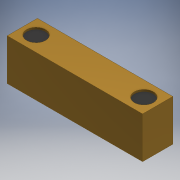
# Autodesk Inventor part: Camera
Saved by Autodesk Inventor 2018 (Build 220112000, 112)
## iProperties
Created: 2018-03-27
Part Number: Camera
Material: Brass, Soft Yellow
Document SubType Name: Modeling
Designer: JARVIS
Mass: 2221.17 g
Surface Area: 296.985 cm^2
Volume: 262.239 cm^3
Density: 8.47 g/cm^3
Appearance: Brass - Satin
Author: JARVIS
Autodesk Inventor part; units mm, degrees
ref_plane "YZ Plane" through (0, 0, 0) normal (1, 0, 0) x (0, 1, 0)
ref_plane "XZ Plane" through (0, 0, 0) normal (0, 1, 0) x (-1, 0, 0)
ref_plane "XY Plane" through (0, 0, 0) normal (0, 0, 1) x (1, 0, 0)
sketch "Sketch1" plane through (0, 0, 0) normal (0, 0, 1) x (1, 0, 0)
  line L0 (-78.5, 17.5) -> (78.5, 17.5)
  line L1 (78.5, 17.5) -> (78.5, -17.5)
  line L2 (78.5, -17.5) -> (-78.5, -17.5)
  line L3 (-78.5, -17.5) -> (-78.5, 17.5)
  point P0 (0, 0)
  point P1 (0, 17.5)
  point P2 (78.5, 0)
  dimension "d0" = 157
  dimension "d1" = 35
  constraints: 8 end point, 2 midpoint, 2 parallel, 1 horizontal, 1 horizontal alignment, 1 perpendicular, 1 vertical alignment
  measures "d0" distance of L0.start L0.end
  measures "d1" distance of L0.end L1.end
extrude "Extrusion1" add sketch "Sketch1" against normal blind 48
sketch "Sketch2" plane through (0, 0, 0) normal (0, 0, 1) x (1, 0, 0)
  circle A0 centre (-62.5, 0) radius 11
  circle A1 centre (62.5, 0) radius 11
  line L0 (-78.5, -17.5) -> (-78.5, 17.5) projected
  point P0 (0, 0)
  dimension "d4" = 22
  dimension "d5" = 22
  dimension "d6" = 125
  dimension "d7" = 16
  constraints: 2 centre point
  measures "d4" diameter of A1
  measures "d5" diameter of A0
  measures "d6" distance of A1.centre A0.centre
  measures "d7" distance from line of A0.centre L0
extrude "Extrusion2" cut sketch "Sketch2" against normal blind 2
equation "\"d5\" = d4"
body "Solid1"
